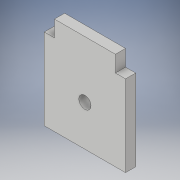
# Autodesk Inventor part: then
Saved by Autodesk Inventor 2019 (Build 230136000, 136)
## iProperties
Created: 2021-01-20
Part Number: then
Material: Generic
Document SubType Name: Modeling
Designer: Admin
Density: 1 g/cm^3
Appearance: Default
Author: Admin
Autodesk Inventor part; units mm, degrees
ref_plane "YZ Plane" through (0, 0, 0) normal (1, 0, 0) x (0, 1, 0)
ref_plane "XZ Plane" through (0, 0, 0) normal (0, 1, 0) x (-1, 0, 0)
ref_plane "XY Plane" through (0, 0, 0) normal (0, 0, 1) x (1, 0, 0)
sketch "Sketch1" plane through (0, 0, 0) normal (0, 0, 1) x (1, 0, 0)
  line L0 (0, 0) -> (0, 20)
  line L1 (20, 20) -> (20, 0)
  line L2 (20, 0) -> (0, 0)
  circle A0 centre (10, 10) radius 1.5
  line L3 (0, 20) -> (2.5, 20)
  line L4 (20, 20) -> (17.5, 20)
  line L5 (17.5, 20) -> (17.5, 24)
  line L6 (17.5, 24) -> (2.5, 24)
  line L7 (2.5, 24) -> (2.5, 20)
  dimension "d0" = 20
  dimension "d1" = 20
  dimension "d2" = 3
  dimension "d3" = 2.5
  dimension "d4" = 2.5
  dimension "d5" = 4
  constraints: 16 end point, 4 perpendicular, 1 centre point, 1 vertical
  measures "d0" distance of L0.start L0.end
  measures "d1" distance of L0.end L1.start
  measures "d2" diameter of A0
  measures "d3" distance of L0.end L3.end
  measures "d4" distance of L1.start L4.end
  measures "d5" distance of L4.end L5.end
extrude "Extrusion1" add sketch "Sketch1" along normal blind 2.5
body "Solid1"
